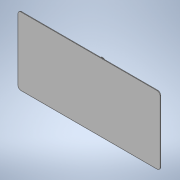
# Autodesk Inventor part: reverse_cat_fire
Saved by Autodesk Inventor 2022 (Build 260153000, 153)
## iProperties
Created: 2024-07-19
Part Number: reverse_cat_fire
Material: Типовые
Document SubType Name: Modeling
Designer: Капустяник Андрей
Density: 1 g/cm^3
Appearance: По умолчанию
Author: Капустяник Андрей
Autodesk Inventor part; units mm, degrees
ref_plane "YZ Plane" through (0, 0, 0) normal (1, 0, 0) x (0, 1, 0)
ref_plane "XZ Plane" through (0, 0, 0) normal (0, 1, 0) x (-1, 0, 0)
ref_plane "XY Plane" through (0, 0, 0) normal (0, 0, 1) x (1, 0, 0)
sketch "Эскиз1" plane through (25.6298, 124.8495, 2.1188) normal (0, 0, 1) x (1, 0, 0)
  line L0 (-43, -80) -> (187, -80)
  line L1 (187, -80) -> (187, 30)
  line L2 (187, 30) -> (-43, 30)
  line L3 (-43, 30) -> (-43, -80)
  line L4 (-43, -80) -> (187, 30) construction
  line L5 (187, -80) -> (-43, 30) construction
  point P0 (-25.6298, -124.8495)
  point P1 (72, -25)
  dimension "d0" = 230
  dimension "d1" = 110
  constraints: 12 end point, 2 midpoint, 2 parallel, 1 horizontal, 1 perpendicular
  measures "d0" distance of L2.end L1.end
  measures "d1" distance of L1.end L0.end
extrude "Выдавливание1" add sketch "Эскиз1" along normal blind 1
fillet "Сопряжение1" radius 5 4 edges at (212.6298, 154.8495, 2.6188) (-17.3702, 154.8495, 2.6188) (-17.3702, 44.8495, 2.6188) (212.6298, 44.8495, 2.6188)
